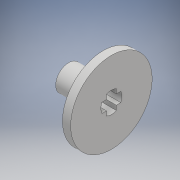
# Autodesk Inventor part: omni-caster-lego-adaptor
Saved by Autodesk Inventor 2018 (Build 220112000, 112)
## iProperties
Created: 2017-11-05
Part Number: omni-caster-lego-adaptor
Material: Generic
Document SubType Name: Modeling
Designer: leo2a
Density: 1 g/cm^3
Appearance: Default
Author: leo2a
Autodesk Inventor part; units mm, degrees
ref_plane "YZ Plane" through (0, 0, 0) normal (1, 0, 0) x (0, 1, 0)
ref_plane "XZ Plane" through (0, 0, 0) normal (0, 1, 0) x (-1, 0, 0)
ref_plane "XY Plane" through (0, 0, 0) normal (0, 0, 1) x (1, 0, 0)
sketch "Sketch3" plane through (0, 0, 0) normal (1, 0, 0) x (0, 1, 0)
  arc A0 (1.2, 2.3065) -> (-1.2, 2.3065) centre (0, 0) ccw
  line L0 (2.6, 1.2) -> (1.2, 1.2)
  line L1 (1.2, 1.2) -> (1.2, 2.6)
  line L2 (-1.2, 2.6) -> (-1.2, 1.2)
  line L3 (-1.2, 1.2) -> (-2.6, 1.2)
  line L4 (-2.6, -1.2) -> (-1.2, -1.2)
  line L5 (-1.2, -1.2) -> (-1.2, -2.6)
  line L6 (1.2, -2.6) -> (1.2, -1.2)
  line L7 (1.2, -1.2) -> (2.6, -1.2)
  arc A1 (-2.3065, 1.2) -> (-2.3065, -1.2) centre (0, 0) ccw
  arc A2 (-1.2, -2.3065) -> (1.2, -2.3065) centre (0, 0) ccw
  arc A3 (2.3065, -1.2) -> (2.3065, 1.2) centre (0, 0) ccw
  circle A4 centre (0, 0) radius 3.175
  dimension "d31" = 360
  dimension "d36" = 6.35
  constraints: 16 end point, 8 point on circle, 8 point on line, 5 centre point, 2 coincident, 1 vertical, 21 other
  measures "d36" diameter of A4
extrude "Extrusion3" add sketch "Sketch3" along normal blind 10.5
sketch "Sketch5" plane through (10.5, 0, 0) normal (1, 0, 0) x (0, 0, -1)
  circle A0 centre (0, 0) radius 2.6
  circle A1 centre (0, 0) radius 10
  dimension "d53" = 20
  constraints: 2 centre point, 1 coincident
  measures "d53" diameter of A1
extrude "Extrusion4" add sketch "Sketch5" against normal blind 2
sketch "Sketch8" plane through (8.5, 0, 0) normal (-1, 0, 0) x (0, 0, 1)
  circle A0 centre (0, 0) radius 5
  circle A1 centre (0, 0) radius 5.5
  circle A2 centre (0, 0) radius 6.5
  circle A3 centre (0, 0) radius 7
  circle A4 centre (0, 0) radius 8
  circle A5 centre (0, 0) radius 8.5
  dimension "d54" = 10
  dimension "d55" = 11
  dimension "d56" = 13
  dimension "d57" = 14
  dimension "d58" = 16
  dimension "d59" = 17
  constraints: 6 centre point, 6 coincident
  measures "d54" diameter of A0
  measures "d55" diameter of A1
  measures "d56" diameter of A2
  measures "d57" diameter of A3
  measures "d58" diameter of A4
  measures "d59" diameter of A5
extrude "Extrusion6" cut sketch "Sketch8" against normal blind 0.1
body "Solid3"
